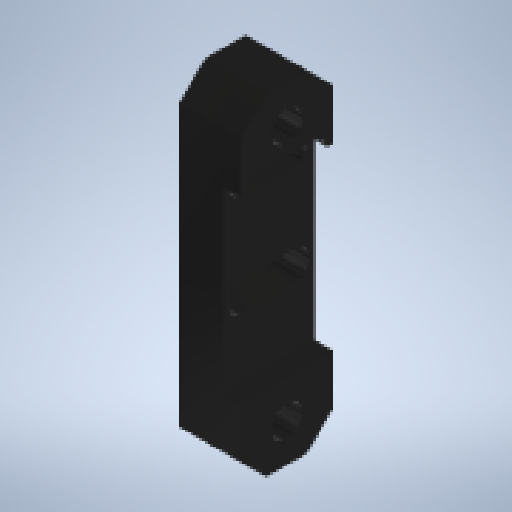
# Autodesk Inventor part: ToolDock_R
Saved by Autodesk Inventor 2023.2 (Build 272271000, 271)
## iProperties
Created: 2022-07-04
Part Number: ToolDock_R
Material: PET Plastic
Document SubType Name: Modeling
Designer: Remo
Density: 1.541 g/cm^3
Appearance: Smooth - Black
Author: Remo
Autodesk Inventor part; units mm, degrees
ref_plane "YZ Plane" through (0, 0, 0) normal (1, 0, 0) x (0, 1, 0)
ref_plane "XZ Plane" through (0, 0, 0) normal (0, 1, 0) x (-1, 0, 0)
ref_plane "XY Plane" through (0, 0, 0) normal (0, 0, 1) x (1, 0, 0)
sketch "Sketch1" plane through (0, 0, 0) normal (1, 0, 0) x (0, 1, 0)
  line L0 (32.5, 9) -> (-32.5, 9)
  line L1 (-32.5, 9) -> (-32.5, -9)
  line L2 (-32.5, -9) -> (32.5, -9)
  line L3 (32.5, -9) -> (32.5, 9)
  line L4 (32.5, 9) -> (-32.5, -9) construction
  line L5 (-32.5, 9) -> (32.5, -9) construction
  circle A0 centre (-25, 0) radius 3
  circle A1 centre (25, 0) radius 3
  line L6 (-3, -5) -> (-3, 5) construction
  line L7 (-6, -5) -> (-6, 5)
  line L8 (0, 5) -> (0, -5)
  arc A2 (-6, -5) -> (0, -5) centre (-3, -5) ccw
  arc A3 (0, 5) -> (-6, 5) centre (-3, 5) ccw
  line L9 (17, -5) -> (17, 5) construction
  line L10 (20, -5) -> (20, 5)
  line L11 (14, 5) -> (14, -5)
  arc A4 (14, -5) -> (20, -5) centre (17, -5) ccw
  arc A5 (20, 5) -> (14, 5) centre (17, 5) ccw
  point P0 (0, 0)
  point P1 (-3, 0)
  point P2 (17, 0)
  point P3 (0, 0)
  dimension "d0" = 25
  dimension "d1" = 50
  dimension "d2" = 65
  dimension "d3" = 6
  dimension "d5" = 20
  dimension "d6" = 10
  dimension "d7" = 3
  dimension "d8" = 18
  dimension "d36" = 3
  constraints: 28 end point, 8 point on circle, 8 tangent, 6 centre point, 5 horizontal alignment, 5 midpoint, 5 parallel, 2 equal radius, 1 horizontal, 1 perpendicular, 1 vertical
  measures "d0" distance of point (0, 0) A0.centre
  measures "d1" distance of A0.centre A1.centre
  measures "d2" distance of L0.start L0.end
  measures "d3" diameter of A0
  measures "d5" distance of point (-3, 0) point (17, 0)
  measures "d6" distance of L6.start L6.end
  measures "d7" radius of A3
  measures "d8" distance of L0.end L1.end
  measures "d36" distance of point (-3, 0) point (0, 0)
extrude "Extrusion1" add sketch "Sketch1" along normal blind 12
sketch "Sketch2" plane through (0, 0, 0) normal (-1, 0, 0) x (0, 0, 1)
  line L0 (9, -32.5) -> (-9, -32.5) projected
  line L1 (9, 32.5) -> (9, -32.5) projected
  line L2 (-9, 32.5) -> (9, 32.5) projected
  line L3 (-9, -32.5) -> (-9, 32.5) projected
  circle A0 centre (0, -25) radius 3 projected
  circle A1 centre (0, 25) radius 3 projected
  arc A2 (-5, 20) -> (-5, 14) centre (-5, 17) ccw projected
  line L4 (5, 20) -> (-5, 20) projected
  arc A3 (5, 14) -> (5, 20) centre (5, 17) ccw projected
  line L5 (-5, 14) -> (5, 14) projected
  line L6 (5, 0) -> (-5, 0) projected
  arc A4 (5, -6) -> (5, 0) centre (5, -3) ccw projected
  line L7 (-5, -6) -> (5, -6) projected
  arc A5 (-5, 0) -> (-5, -6) centre (-5, -3) ccw projected
  line L8 (5, 17) -> (-5, 17) construction
  line L9 (5, 15.25) -> (-5, 15.25)
  line L10 (-5, 18.75) -> (5, 18.75)
  arc A6 (5, 15.25) -> (5, 18.75) centre (5, 17) ccw
  arc A7 (-5, 18.75) -> (-5, 15.25) centre (-5, 17) ccw
  line L11 (5, -3) -> (-5, -3) construction
  line L12 (5, -4.75) -> (-5, -4.75)
  line L13 (-5, -1.25) -> (5, -1.25)
  arc A8 (5, -4.75) -> (5, -1.25) centre (5, -3) ccw
  arc A9 (-5, -1.25) -> (-5, -4.75) centre (-5, -3) ccw
  point P0 (0, 0)
  point P1 (0, 17)
  point P2 (0, -3)
  dimension "d11" = 3.5
  constraints: 16 end point, 8 point on circle, 8 tangent, 4 centre point, 3 parallel, 2 midpoint, 1 equal radius, 1 horizontal
  measures "d11" distance between parallel lines of L10 L9
extrude "Extrusion2" add sketch "Sketch2" against normal blind 3 contours L4 A3 L5 A2 | A4 L7 A5 L6
chamfer "Chamfer1" distance 5 angle 45 4 edges at (6, -32.5, 9) (6, -32.5, -9) (6, 32.5, -9) (6, 32.5, 9)
sketch "Sketch3" plane through (0, -27.5, 9) normal (0, 0, 1) x (1, 0, 0)
  line L0 (0, 55) -> (12, 55) projected
  line L1 (0, 55) -> (0, 0) projected
  line L2 (12, 0) -> (0, 0) projected
  line L3 (12, 55) -> (12, 0) projected
  line L4 (12, 10) -> (8.5, 10)
  line L5 (8.5, 10) -> (8.5, 45)
  line L6 (8.5, 45) -> (12, 45)
  line L7 (12, 45) -> (12, 10)
  line L8 (12, 10) -> (8.5, 45) construction
  line L9 (8.5, 10) -> (12, 45) construction
  point P0 (0, 27.5)
  point P1 (10.25, 27.5)
  point P2 (0, 27.5)
  point P3 (12, 10)
  dimension "d17" = 35
  dimension "d18" = 3.5
  constraints: 12 end point, 3 midpoint, 2 parallel, 1 horizontal, 1 horizontal alignment, 1 perpendicular, 1 vertical alignment
  measures "d17" distance of L4.end L5.end
  measures "d18" distance of L5.end L6.end
extrude "Extrusion3" cut sketch "Sketch3" against normal through all contours L3 L4 L5 L6
equation "\"d1\" = 2 * d0"
equation "\"d36\" = d7"
body "Solid1"
